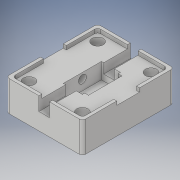
# Autodesk Inventor part: Enclosure_Bottom V2D5
Saved by Autodesk Inventor 2017 (Build 210142000, 142)
## iProperties
Created: 2017-11-29
Part Number: Enclosure_Bottom V2D5
Material: Generic
Document SubType Name: Modeling
Designer: Tripl_000
Density: 1 g/cm^3
Appearance: Default
Author: Tripl_000
Autodesk Inventor part; units mm, degrees
ref_plane "YZ Plane" through (0, 0, 0) normal (1, 0, 0) x (0, 1, 0)
ref_plane "XZ Plane" through (0, 0, 0) normal (0, 1, 0) x (-1, 0, 0)
ref_plane "XY Plane" through (0, 0, 0) normal (0, 0, 1) x (1, 0, 0)
sketch "Sketch1" plane through (0, 0, 0) normal (0, 1, 0) x (-1, 0, 0)
  line L0 (-25, 30) -> (25, 30)
  line L1 (25, 30) -> (25, -30)
  line L2 (25, -30) -> (-25, -30)
  line L3 (-25, -30) -> (-25, 30)
  line L4 (-25, 30) -> (25, -30) construction
  line L5 (25, 30) -> (-25, -30) construction
  point P0 (0, 0)
  dimension "d0" = 50
  dimension "d1" = 60
  constraints: 12 end point, 2 midpoint, 2 parallel, 1 horizontal, 1 perpendicular
  measures "d0" distance of L1.end L2.end
  measures "d1" distance of L0.end L1.end
extrude "Extrusion1" add sketch "Sketch1" along normal blind 20
sketch "Sketch2" plane through (-25, 0, 30) normal (0, 0, 1) x (1, 0, 0)
  line L0 (0, 20) -> (50, 20) projected
  line L1 (21.5, 20) -> (28.5, 20)
  line L2 (28.5, 20) -> (28.5, 13)
  line L3 (28.5, 13) -> (21.5, 13)
  line L4 (21.5, 13) -> (21.5, 20)
  line L5 (0, 0) -> (0, 20) projected
  point P0 (25, 0)
  dimension "d4" = 7
  dimension "d5" = 7
  dimension "d6" = 21.5
  constraints: 8 end point, 2 parallel, 1 horizontal, 1 perpendicular, 1 point on line
  measures "d4" distance between parallel lines of L2 L4
  measures "d5" distance between parallel lines of L0 L3
  measures "d6" distance between parallel lines of L4 L5
sketch "Sketch3" plane through (0, 20, 0) normal (0, 1, 0) x (1, 0, 0)
  line L0 (-8.5, 7.5) -> (8.5, 7.5)
  line L1 (8.5, 7.5) -> (8.5, -7.5)
  line L2 (8.5, -7.5) -> (-8.5, -7.5)
  line L3 (-8.5, -7.5) -> (-8.5, 7.5)
  line L4 (-8.5, 7.5) -> (8.5, -7.5) construction
  line L5 (8.5, 7.5) -> (-8.5, -7.5) construction
  point P0 (0, 0)
  dimension "d7" = 17
  dimension "d8" = 15
  constraints: 12 end point, 2 midpoint, 2 parallel, 1 horizontal, 1 perpendicular
  measures "d7" distance of L0.start L0.end
  measures "d8" distance between parallel lines of L2 L0
shell "Shell1" thickness 2 removed faces 1 at (-8.3333, 20, -10)
sketch "Sketch4" plane through (-23, 2, 28) normal (0, 1, 0) x (1, 0, 0)
  line L0 (0, 0) -> (0, 56) projected
  line L1 (46, 56) -> (46, 0) projected
  line L2 (0, 56) -> (46, 56)
  line L3 (46, 56) -> (46, 0)
  line L4 (46, 0) -> (0, 0)
  line L5 (0, 0) -> (0, 56)
  point P0 (23, 28)
  constraints: 8 end point, 2 parallel, 1 horizontal, 1 perpendicular
extrude "Extrusion2" add sketch "Sketch4" along normal blind 15.5
extrude "Extrusion3" cut sketch "Sketch3" against normal blind 13
extrude "Extrusion4" cut sketch "Sketch2" against normal through all
sketch "Sketch5" plane through (-23, 17.5, 28) normal (0, 1, 0) x (1, 0, 0)
  circle A0 centre (5.5, 50.5) radius 3.683
  line L0 (-27.6389, 28) -> (76.1675, 28)
  line L1 (23, 61.4826) -> (23, -6.2799)
  circle A1 centre (40.5, 50.5) radius 3.683
  circle A2 centre (5.5, 5.5) radius 3.683
  circle A3 centre (40.5, 5.5) radius 3.683
  point P0 (23, 28)
  dimension "d16" = 22.5
  dimension "d17" = 17.5
  dimension "d18" = 7.366
  constraints: 4 centre point, 4 end point, 3 symmetric about line, 1 horizontal, 1 vertical, 3 other
  measures "d16" vertical distance of point (23, 28) A0.centre
  measures "d17" horizontal distance of point (23, 28) A0.centre
  measures "d18" diameter of A0
fillet "Fillet1" radius 2 8 edges at (25, 10, 30) (25, 10, -30) (-25, 10, 30) (-25, 10, -30) (-23, 18.75, -28) (23, 18.75, -28) (-23, 18.75, 28) (23, 18.75, 28)
extrude "Extrusion6" cut sketch "Sketch5" against normal through all
ref_plane "Work Plane1" through (0, 17.5, 0) normal (0, 1, 0) x (1, 0, 0)
sketch "Sketch6" plane through (0, 17.5, 0) normal (0, 1, 0) x (1, 0, 0)
  line L0 (-12.5, 12.5) -> (12.5, 12.5)
  line L1 (12.5, 12.5) -> (12.5, -12.5)
  line L2 (12.5, -12.5) -> (-12.5, -12.5)
  line L3 (-12.5, -12.5) -> (-12.5, 12.5)
  line L4 (-12.5, 12.5) -> (12.5, -12.5) construction
  line L5 (12.5, 12.5) -> (-12.5, -12.5) construction
  point P0 (0, 0)
  dimension "d25" = 25
  dimension "d26" = 25
  constraints: 12 end point, 2 midpoint, 2 parallel, 1 horizontal, 1 perpendicular
  measures "d25" distance of L0.end L1.end
  measures "d26" distance of L0.start L0.end
sketch "Sketch7" plane through (25, 0, 28) normal (1, 0, 0) x (0, 0, -1)
  line L0 (54, 20) -> (2, 20) projected
  line L1 (35.5, 20) -> (20.5, 20)
  line L2 (20.5, 20) -> (20.5, 17.5)
  line L3 (20.5, 17.5) -> (35.5, 17.5)
  line L4 (35.5, 17.5) -> (35.5, 20)
  line L5 (-2, 20) -> (-2, 0) projected
  point P0 (28, 0)
  dimension "d27" = 22.5
  dimension "d28" = 15
  dimension "d29" = 2.5
  constraints: 8 end point, 2 parallel, 1 horizontal, 1 perpendicular, 1 point on line
  measures "d27" distance between parallel lines of L5 L2
  measures "d28" distance between parallel lines of L2 L4
  measures "d29" distance between parallel lines of L0 L3
extrude "Extrusion7" cut sketch "Sketch7" against normal through all
extrude "Extrusion8" cut sketch "Sketch6" against normal up to surface (10.5 mm away)
sketch "Sketch8" plane through (-12.5, 7, -12.5) normal (1, 0, 0) x (0, 0, -1)
  circle A0 centre (-12.5, 6.6382) radius 2.6
  point P0 (-12.5, -7)
  dimension "d38" = 5.2
  constraints: 1 centre point
  measures "d38" diameter of A0
extrude "Extrusion9" cut sketch "Sketch8" against normal blind 6.7
sketch "Sketch9" plane through (-19.2, 13.6382, 0) normal (1, 0, 0) x (0, 0, -1)
  circle A0 centre (0, 0) radius 3.2
  point P0 (0, -13.6382)
  dimension "d41" = 6.4
  constraints: 1 centre point
  measures "d41" diameter of A0
extrude "Extrusion10" cut sketch "Sketch9" against normal through all
sketch "Sketch10" plane through (-23, 17.5, 28) normal (0, 1, 0) x (1, 0, 0)
  line L0 (10.5, 40.5) -> (10.5, 15.5) projected
  line L1 (10.5, 40.5) -> (19.5, 40.5) projected
  line L2 (10.5, 15.5) -> (18, 15.5)
  line L3 (18, 40.5) -> (10.5, 40.5)
  line L4 (10.5, 31.375) -> (18, 31.375)
  line L5 (10.5, 24.625) -> (18, 24.625)
  line L6 (18, 15.5) -> (18, 24.625)
  line L7 (18, 31.375) -> (18, 40.5)
  line L8 (10.5, 40.5) -> (10.5, 31.375)
  line L9 (10.5, 24.625) -> (10.5, 15.5)
  point P0 (23, 28)
  dimension "d45" = 6.75
  dimension "d46" = 9.125
  constraints: 16 end point, 6 perpendicular, 5 parallel, 1 horizontal, 1 point on line
  measures "d45" distance between parallel lines of L4 L5
  measures "d46" distance between parallel lines of L4 L1
extrude "Extrusion11" add sketch "Sketch10" against normal up to surface (10.5 mm away)
sketch "Sketch11" plane through (0, 7, 0) normal (0, 1, 0) x (1, 0, 0)
  line L0 (-5, -12.5) -> (12.5, -12.5) projected
  line L1 (12.5, 12.5) -> (-5, 12.5) projected
  line L2 (12.5, -12.5) -> (10, -12.5)
  line L3 (10, -12.5) -> (10, 12.5)
  line L4 (10, 12.5) -> (12.5, 12.5)
  line L5 (12.5, 12.5) -> (12.5, -12.5)
  point P0 (0, 0)
  dimension "d49" = 2.5
  constraints: 8 end point, 2 parallel, 1 horizontal, 1 perpendicular, 1 point on line
  measures "d49" distance between parallel lines of L5 L3
extrude "Extrusion12" cut sketch "Sketch11" against normal blind 2.2
sketch "Sketch12" plane through (-12.5, 7, 3.375) normal (1, 0, 0) x (0, 0, -1)
  line L0 (6.75, 0) -> (0, 0) projected
  line L1 (0, 10.5) -> (0, 0) projected
  line L2 (6.75, 0) -> (0, 0)
  line L3 (0, 0) -> (0, 3)
  line L4 (0, 3) -> (6.75, 3)
  line L5 (6.75, 3) -> (6.75, 0)
  point P0 (3.375, -7)
  dimension "d56" = 3
  constraints: 8 end point, 2 parallel, 1 horizontal, 1 perpendicular, 1 point on line
  measures "d56" distance between parallel lines of L0 L4
extrude "Extrusion13" add sketch "Sketch12" along normal up to surface (7.5 mm away)
sketch "Sketch13" plane through (-23, 17.5, 28) normal (0, 1, 0) x (1, 0, 0)
  line L0 (10.5, 31.375) -> (18, 31.375) projected
  line L1 (18, 24.625) -> (10.5, 24.625) projected
  line L2 (18, 31.375) -> (10.5, 31.375)
  line L3 (10.5, 31.375) -> (10.5, 24.625)
  line L4 (10.5, 24.625) -> (18, 24.625)
  line L5 (18, 24.625) -> (18, 31.375)
  point P0 (23, 28)
  constraints: 8 end point, 2 parallel, 1 horizontal, 1 perpendicular
extrude "Extrusion14" add sketch "Sketch13" against normal up to surface (7.5 mm away)
sketch "Sketch14" plane through (-5, 17.5, 12.5) normal (1, 0, 0) x (0, 0, -1)
  circle A0 centre (12.5, -3.8618) radius 2.6 projected
  circle A1 centre (12.5, -3.8618) radius 2.6
  point P0 (12.5, -17.5)
  constraints: 1 centre point, 1 coincident
extrude "Extrusion15" cut sketch "Sketch14" against normal blind 6.7
sketch "Sketch15" plane through (-19.2, 13.6382, 0) normal (-1, 0, 0) x (0, 0, 1)
  circle A0 centre (0, 0) radius 3.2
  point P0 (0, -13.6382)
  constraints: 1 centre point
extrude "Extrusion16" cut sketch "Sketch15" against normal up to surface (7.5 mm away)
sketch "Sketch16" plane through (-23, 17.5, 28) normal (0, 1, 0) x (1, 0, 0)
  line L0 (35.5, 40.5) -> (35.5, 15.5) projected
  line L1 (35.5, 15.5) -> (26.5, 15.5) projected
  line L2 (35.5, 40.5) -> (30.5, 40.5)
  line L3 (30.5, 40.5) -> (30.5, 15.5)
  line L4 (30.5, 15.5) -> (35.5, 15.5)
  line L5 (35.5, 15.5) -> (35.5, 40.5)
  point P0 (23, 28)
  dimension "d73" = 5
  constraints: 8 end point, 2 parallel, 1 horizontal, 1 perpendicular, 1 point on line
  measures "d73" distance between parallel lines of L0 L3
extrude "Extrusion17" add sketch "Sketch16" against normal up to surface (12.7 mm away)
sketch "Sketch17" plane through (-23, 17.5, 28) normal (0, 1, 0) x (1, 0, 0)
  line L0 (26.5, 40.5) -> (30.5, 40.5) projected
  line L1 (30.5, 40.5) -> (33, 40.5)
  line L2 (33, 40.5) -> (33, 15.5)
  line L3 (33, 15.5) -> (30.5, 15.5)
  line L4 (30.5, 15.5) -> (30.5, 40.5)
  point P0 (23, 28)
  dimension "d76" = 2.5
  constraints: 8 end point, 2 parallel, 1 horizontal, 1 perpendicular
  measures "d76" distance between parallel lines of L2 L4
extrude "Extrusion18" cut sketch "Sketch17" against normal blind 12.7
sketch "Sketch18" plane through (-23, 17.5, 28) normal (0, 1, 0) x (1, 0, 0)
  line L0 (26.5, 40.5) -> (33, 40.5) projected
  line L1 (30.5, 15.5) -> (30.5, 40.5) projected
  line L2 (33, 40.5) -> (30.5, 40.5)
  line L3 (30.5, 15.5) -> (33, 15.5)
  line L4 (30.5, 39) -> (33, 39)
  line L5 (30.5, 17) -> (33, 17)
  line L6 (33, 40.5) -> (33, 15.5) projected
  line L7 (33, 15.5) -> (33, 17)
  line L8 (33, 39) -> (33, 40.5)
  line L9 (30.5, 40.5) -> (30.5, 39)
  line L10 (30.5, 17) -> (30.5, 15.5)
  point P0 (23, 28)
  dimension "d79" = 22
  dimension "d80" = 1.5
  constraints: 16 end point, 6 parallel, 3 perpendicular, 1 horizontal, 1 point on line
  measures "d79" distance between parallel lines of L5 L4
  measures "d80" distance between parallel lines of L3 L5
extrude "Extrusion19" add sketch "Sketch18" against normal up to surface (12.7 mm away) contours L0 L6 L4 L1 | L5 L6 L3 L1
sketch "Sketch19" plane through (-3.5, 13, -30) normal (0, 1, 0) x (1, 0, 0)
  line L0 (0, -17.5) -> (0, 0) projected
  line L1 (7, -60) -> (7, -42.5) projected
  line L2 (0, 0) -> (7, 0)
  line L3 (7, 0) -> (7, -60)
  line L4 (7, -60) -> (0, -60)
  line L5 (0, -60) -> (0, 0)
  point P0 (3.5, -30)
  constraints: 8 end point, 2 parallel, 1 horizontal, 1 perpendicular
extrude "Extrusion20" cut sketch "Sketch19" against normal blind 1.96
body "Solid1"
